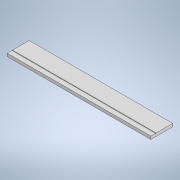
# Autodesk Inventor part: big bourd
Saved by Autodesk Inventor 2021 (Build 250183000, 183)
## iProperties
Created: 2021-07-05
Part Number: big bourd
Material: Generic
Document SubType Name: Modeling
Designer: newic
Density: 1 g/cm^3
Appearance: Default
Author: newic
Autodesk Inventor part; units mm, degrees
ref_plane "YZ Plane" through (0, 0, 0) normal (1, 0, 0) x (0, 1, 0)
ref_plane "XZ Plane" through (0, 0, 0) normal (0, 1, 0) x (-1, 0, 0)
ref_plane "XY Plane" through (0, 0, 0) normal (0, 0, 1) x (1, 0, 0)
sketch "Sketch1" plane through (0, 0, 0) normal (1, 0, 0) x (0, 1, 0)
  line L0 (0, 0) -> (19.05, 0)
  line L1 (19.05, 0) -> (19.05, -139.7)
  line L2 (19.05, -139.7) -> (0, -139.7)
  line L3 (0, -139.7) -> (0, 0)
  dimension "d0" = 19.05
  dimension "d1" = 139.7
  constraints: 8 end point, 2 parallel, 1 horizontal, 1 perpendicular
  measures "d0" distance of L1.end L2.end
  measures "d1" distance of L0.end L1.end
extrude "Extrusion1" add sketch "Sketch1" along normal blind 914.4
sketch "Sketch2" plane through (0, 0, 0) normal (-1, 0, 0) x (0, 0, 1)
  line L0 (0, 7.6875) -> (-31.75, 7.6875)
  line L1 (-31.75, 7.6875) -> (-31.75, 36.5157)
  line L2 (-139.7, 19.05) -> (0, 19.05) projected
  line L3 (-139.7, 13.97) -> (0, 13.97)
  line L4 (-31.75, 13.97) -> (-23.9508, 35.3981)
  line L5 (-31.75, 13.97) -> (-38.1681, 31.6036)
  point P0 (0, 0)
  point P1 (-29.901, 19.05)
  point P2 (-33.599, 19.05)
  dimension "d4" = 31.75
  dimension "d5" = 5.08
  dimension "d6" = 20
  dimension "d7" = 20
  constraints: 10 end point, 2 point on line, 1 horizontal, 1 parallel, 1 vertical
  measures "d4" distance of L0.start L0.end
  measures "d5" distance between parallel lines of L2 L3
  measures "d6" angle of L1 L5
  measures "d7" angle of L4 L1
extrude "Extrusion2" cut sketch "Sketch2" against normal through all
body "Solid1"
